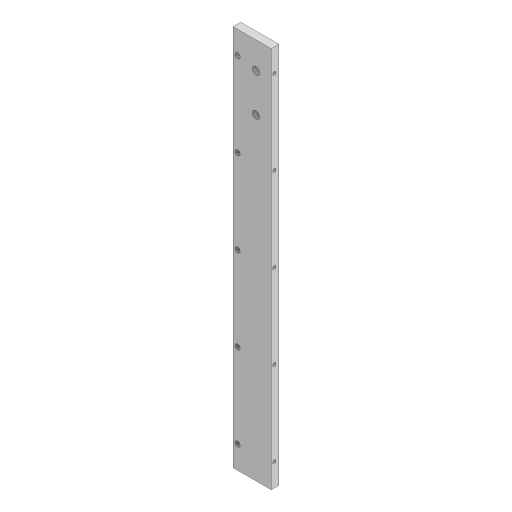
# Autodesk Inventor part: Platte-1
Saved by Autodesk Inventor 2024.3 (Build 283343000, 343)
## iProperties
Created: 2025-05-16
Part Number: Platte-1
Material: Generisch
Document SubType Name: Modeling
Designer: Demir
Density: 1 g/cm^3
Appearance: Vorgabe
Author: Demir
Autodesk Inventor part; units mm, degrees
ref_plane "YZ Plane" through (0, 0, 0) normal (1, 0, 0) x (0, 1, 0)
ref_plane "XZ Plane" through (0, 0, 0) normal (0, 1, 0) x (-1, 0, 0)
ref_plane "XY Plane" through (0, 0, 0) normal (0, 0, 1) x (1, 0, 0)
sketch "Skizze1" plane through (0, 0, 0) normal (0, 0, 1) x (1, 0, 0)
  line L0 (-25, 5) -> (25, 5)
  line L1 (25, 5) -> (25, -5)
  line L2 (25, -5) -> (-25, -5)
  line L3 (-25, -5) -> (-25, 5)
  line L4 (-25, 5) -> (25, -5) construction
  line L5 (25, 5) -> (-25, -5) construction
  point P0 (0, 0)
  dimension "d0" = 50
  dimension "d1" = 10
  constraints: 12 end point, 2 midpoint, 2 parallel, 1 horizontal, 1 perpendicular
  measures "d0" distance of L0.start L0.end
  measures "d1" distance of L2.end L0.start
extrude "Extrusion1" add sketch "Skizze1" along normal mid plane 500
sketch "Skizze2" plane through (-25, 5, 250) normal (0, 1, 0) x (1, 0, 0)
  line L0 (0, 500) -> (0, 0) projected
  line L1 (50, 0) -> (0, 0) projected
  line L2 (50, 500) -> (50, 0) projected
  line L3 (0, 500) -> (50, 500) projected
  point P0 (25, 250)
  point P1 (30, 35)
  point P2 (25, 0)
  point P3 (30, 85)
  dimension "d28" = 30
  dimension "d29" = 35
  dimension "d30" = 50
  constraints: 1 midpoint, 1 vertical alignment
  measures "d28" distance from line of point (30, 35) L0
  measures "d29" distance from line of point (30, 35) L1
  measures "d30" distance of point (30, 85) point (30, 35)
hole "Bohrung1" at (5, 5, 215) at (5, 5, 165) direction (0, -1, 0) diameter 8.5 depth 20 tip angle 118
sketch "Skizze3" plane through (-25, 5, 250) normal (0, 1, 0) x (1, 0, 0)
  circle A0 centre (30, 85) radius 4.25 projected
  circle A1 centre (30, 35) radius 4.25 projected
  line L0 (0, 500) -> (0, 0) projected
  line L1 (50, 0) -> (0, 0) projected
  line L2 (50, 500) -> (50, 0) projected
  line L3 (0, 500) -> (50, 500) projected
  point P0 (25, 250)
  point P1 (6, 250)
  dimension "d14" = 6
  constraints: 1 horizontal alignment
  measures "d14" distance from line of point (6, 250) L0
hole "Bohrung2" at (-19, 5, 0) direction (0, -1, 0) diameter 5.5 depth 32.3 tip angle 118 counterbore diameter 10 counterbore depth 5
pattern_linear "Rechteckige Anordnung1" count 3 spacing 110 along (0, 0, 1) count 3 spacing 110 along (0, 0, -1) of "Bohrung2"
sketch "Skizze4" plane through (25, 5, 250) normal (1, 0, 0) x (0, 0, -1)
  line L0 (500, 0) -> (0, 0) projected
  line L1 (0, -10) -> (0, 0) projected
  line L2 (500, -10) -> (0, -10) projected
  line L3 (500, 0) -> (500, -10) projected
  point P0 (250, -5)
  point P1 (250, -6)
  dimension "d55" = 6
  constraints: 1 vertical alignment
  measures "d55" distance from line of point (250, -6) L0
hole "Bohrung3" at (25, -1, 0) direction (-1, 0, 0) diameter 4.134 depth 14.2 tip angle 118 thread size "M5x0.8" class "6H" standard "ISO Metric profile"
pattern_linear "Rechteckige Anordnung2" count 3 spacing 110 along (0, 0, -1) count 3 spacing 110 along (0, 0, 1) of "Bohrung3"
sketch "Skizze5" plane through (0, 0, -250) normal (0, 0, -1) x (-1, 0, 0)
  line L0 (-25, -5) -> (25, -5) projected
  line L1 (25, -5) -> (25, 5) projected
  line L2 (25, 5) -> (-25, 5) projected
  line L3 (-25, 5) -> (-25, -5) projected
  point P0 (0, 0)
  point P1 (19, -1)
  dimension "d44" = 6
  dimension "d56" = 4
  measures "d44" distance from line of point (19, -1) L1
  measures "d56" distance from line of point (19, -1) L0
hole "Bohrung4" at (-19, -1, -250) direction (0, 0, 1) diameter 4.134 depth 20 tip angle 118 thread size "M5x0.8" class "6H" standard "ISO Metric profile"
chamfer "Fasen1" distance 0.5 angle 45 1 edges at (-19, -3.067, -250)
chamfer "Fasen2" distance 0.5 angle 45 5 edges at (-19, 5, -225) (-19, 5, -115) (-19, 5, -5) (-19, 5, 105) (-19, 5, 215)
chamfer "Fasen3" distance 0.5 angle 45 4 edges at (5, 5, 160.75) (5, -5, 160.75) (5, 5, 210.75) (5, -5, 210.75)
chamfer "Fasen4" distance 0.5 angle 45 5 edges at (-19, -5, -222.75) (-19, -5, -112.75) (-19, -5, -2.75) (-19, -5, 107.25) (-19, -5, 217.25)
